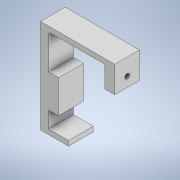
# Autodesk Inventor part: agarre motor
Saved by Autodesk Inventor 2021 (Build 250183000, 183)
## iProperties
Created: 2021-05-13
Part Number: agarre motor
Material: Genérico
Document SubType Name: Modeling
Designer: orgyn
Density: 1 g/cm^3
Appearance: Valor por defecto
Author: orgyn
Autodesk Inventor part; units mm, degrees
ref_plane "YZ Plane" through (0, 0, 0) normal (1, 0, 0) x (0, 1, 0)
ref_plane "XZ Plane" through (0, 0, 0) normal (0, 1, 0) x (-1, 0, 0)
ref_plane "XY Plane" through (0, 0, 0) normal (0, 0, 1) x (1, 0, 0)
sketch "Boceto1" plane through (0, 0, 0) normal (0, 1, 0) x (-1, 0, 0)
  line L0 (0, 0) -> (22, 0)
  line L1 (22, 0) -> (22, -15)
  line L2 (22, -15) -> (0, -15)
  line L3 (0, -15) -> (-12, -15)
  line L4 (-12, -15) -> (-12, 0)
  line L5 (-12, 0) -> (0, 0)
  dimension "d15" = 12
  constraints: 12 end point, 2 horizontal, 2 perpendicular, 1 collinear, 1 parallel
  measures "d15" distance of L2.end L3.end
extrude "Extrusión1" add sketch "Boceto1" along normal blind 3
sketch "Boceto3" plane through (0, 3, 0) normal (0, 1, 0) x (1, 0, 0)
  line L0 (-22, 15) -> (-22, 0) projected
  line L1 (-22, 15) -> (-27, 15)
  line L2 (-27, 15) -> (-27, 0)
  line L3 (-27, 0) -> (-22, 0)
  line L4 (-22, 0) -> (-22, 15)
  point P0 (0, 0)
  dimension "d4" = 5
  constraints: 8 end point, 2 parallel, 1 horizontal, 1 perpendicular
  measures "d4" distance of L3.end L2.end
extrude "Extrusión2" add sketch "Boceto3" against normal blind 57
sketch "Boceto4" plane through (-22, -54, 0) normal (1, 0, 0) x (0, 0, -1)
  point P0 (0, 54)
sketch "Boceto5" plane through (-22, -54, 0) normal (1, 0, 0) x (0, 0, -1)
  line L0 (0, 57) -> (0, 0) projected
  line L1 (15, 57) -> (15, 0) projected
  line L2 (0, 0) -> (15, 0)
  line L3 (15, 0) -> (15, 3.0333)
  line L4 (15, 3.0333) -> (0, 3.0333)
  line L5 (0, 3.0333) -> (0, 0)
  point P0 (0, 54)
  constraints: 8 end point, 2 parallel, 1 horizontal, 1 perpendicular, 1 point on line
extrude "Extrusión3" add sketch "Boceto5" along normal blind 12
sketch "Boceto7" plane through (12, 0, 0) normal (1, 0, 0) x (0, 0, -1)
  line L0 (0, 0) -> (0, -50.9667) projected
  line L1 (0, 3) -> (0, 0)
  line L2 (0, 0) -> (0, -7)
  line L3 (0, -7) -> (10.8666, -7)
  line L4 (0, -7) -> (0, -13)
  line L5 (0, -13) -> (15, -13)
  line L6 (15, 0) -> (15, -50.9667) projected
  line L7 (15, 3) -> (15, -54) projected
  line L8 (15, 3) -> (15, -13)
  line L9 (15, 3) -> (0, 3) projected
  line L10 (15, 3) -> (0, 3)
  line L11 (0, 3) -> (0, -13)
  line L12 (0, -7) -> (15, -7)
  circle A0 centre (7.5, -7) radius 1.5
  dimension "d16" = 7
  dimension "d17" = 6
  dimension "d18" = 3
  constraints: 18 end point, 5 point on line, 3 perpendicular, 2 collinear, 1 centre point, 1 midpoint, 1 vertical
  measures "d16" distance of L0.start L2.end
  measures "d17" distance of L2.end L4.end
  measures "d18" diameter of A0
extrude "Extrusión5" add sketch "Boceto7" along normal blind 6 contours L1 L9 L7 L6 L12 L3 A0 L0 | L3 A0 L12 L6 L5 L0
sketch "Boceto8" plane through (-22, 0, 0) normal (1, 0, 0) x (0, 0, -1)
  line L0 (15, -50.9667) -> (0, -50.9667) projected
  line L1 (0, -50.9667) -> (0, -40.9667)
  line L2 (0, 0) -> (0, -50.9667) projected
  line L3 (0, -40.9667) -> (0, -38.9667)
  line L4 (0, -38.9667) -> (15, -38.9667)
  line L5 (15, 0) -> (15, -50.9667) projected
  line L6 (0, -40.9667) -> (15, -40.9667)
  line L7 (15, -40.9667) -> (15, -38.9667)
  dimension "d21" = 10
  dimension "d22" = 2
  constraints: 10 end point, 3 point on line, 2 perpendicular, 1 horizontal
  measures "d21" distance of L0.end L1.end
  measures "d22" distance of L1.end L3.end
extrude "Extrusión6" add sketch "Boceto8" along normal blind 6 contours L6 L2 L4 L5
sketch "Boceto9" plane through (-22, -38.9667, 0) normal (0, 1, 0) x (1, 0, 0)
  line L0 (0, 0) -> (0, 15) projected
  line L1 (0, 0) -> (0, 15)
  line L2 (6, 15) -> (6, 0) projected
  line L3 (0, 15) -> (6, 15)
  line L4 (6, 15) -> (6, 0)
  line L5 (0, 15) -> (0, 0) projected
  line L6 (6, 0) -> (0, 0)
  point P0 (22, 0)
  constraints: 8 end point, 3 perpendicular, 1 collinear
extrude "Extrusión7" add sketch "Boceto9" along normal blind 18
